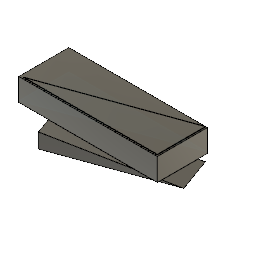
Pill holder for dispense v1 (Autodesk Fusion 360 design; units mm, degrees)
Autodesk Fusion 360 part; units mm, degrees
sketch "Sketch3" plane through (0, 0, 0) normal (0, 0, 1) x (1, 0, 0) in component "Pill Holder "
  line L0 (0, -3.5074) -> (3, -3.5074)
  line L1 (3, -3.5074) -> (3, 110.4926)
  line L2 (3, 110.4926) -> (0, 110.4926)
  line L3 (0, 110.4926) -> (0, -3.5074)
  dimension "d20" = 114
  dimension "d21" = 3
  constraint horizontal L0
  constraint vertical L1
  constraint horizontal L2
  constraint vertical L3
  measures "d20" distance of L0.end L1.end
  measures "d21" distance of L0.start L0.end
extrude "Extrude6" add sketch "Sketch3" along normal blind 50 makes body 1 in component "Pill Holder "
sketch "Sketch4" plane through (0, 0, 0) normal (-1, 0, 0) x (0, -1, 0) in component "Pill Holder "
  line L0 (-110.4926, 0) -> (3.5074, 0)
  line L1 (3.5074, 0) -> (3.5074, 50)
  line L2 (3.5074, 50) -> (-110.4926, 50)
  line L3 (-110.4926, 50) -> (-110.4926, 0)
  line L4 (0.5074, 3) -> (-107.4926, 3)
  line L5 (-107.4926, 3) -> (-107.4926, 47)
  line L6 (-107.4926, 47) -> (0.5074, 47)
  line L7 (0.5074, 47) -> (0.5074, 3)
  dimension "d24" = 3
  dimension "d25" = 3
  dimension "d26" = 3
  dimension "d27" = 3
  constraint horizontal L4
  constraint vertical L5
  constraint horizontal L6
  constraint vertical L7
  measures "d24" distance of L0 L4
  measures "d25" distance of L2 L6
  measures "d26" distance of L1 L7
  measures "d27" distance of L3 L5
extrude "Extrude7" add sketch "Sketch4" along normal blind 304 bodies 1 in component "Pill Holder "
extrude "Extrude8" cut 1 faces at (-201.6667, 110.4926, 16.6667) along direction (0, -1, 0) blind 3 on bodies 1 bodies 1 in component "Pill Holder "
sketch "Sketch5" plane through (0, 0, 3) normal (0, 0, 1) x (-1, 0, 0) in component "Pill Holder "
  line L0 (0, 0.5074) -> (0, -107.4926)
  line L1 (0, -107.4926) -> (304, -107.4926)
  line L2 (304, -107.4926) -> (304, 0.5074)
  line L3 (304, 0.5074) -> (0, 0.5074)
  line L4 (-3, -107.4926) -> (304, -107.4926)
  line L5 (304, -107.4926) -> (304, 3.5074)
  line L6 (304, 3.5074) -> (-3, 3.5074)
  line L7 (-3, 3.5074) -> (-3, -107.4926)
  line L8 (0, -107.4926) -> (0, 0.5074)
  line L9 (0, 0.5074) -> (304, 0.5074)
  line L10 (304, 0.5074) -> (304, -107.4926)
  line L11 (304, -107.4926) -> (0, -107.4926)
  line L12 (304, 3.5074) -> (-3, -107.4926)
  constraint coincident L5.end L6.start
  constraint coincident L4.start L7.end
extrude "Extrude11" add sketch "Sketch5" along normal blind 48 contours L0 L3 L8 L9 L12 bodies 1 in component "Pill Holder "
sketch "Sketch6" plane through (-304, 0, 0) normal (-1, 0, 0) x (0, -1, 0) in component "Pill Holder "
  line L0 (-107.4926, 50) -> (-107.4926, 47)
  line L1 (-107.4926, 47) -> (0.5074, 47)
  line L2 (0.5074, 3) -> (-107.4926, 3)
  line L3 (-107.4926, 0) -> (3.5074, 0)
  line L4 (3.5074, 0) -> (3.5074, 50)
  line L5 (3.5074, 50) -> (-107.4926, 50)
  line L6 (3.5074, 9.4187) -> (-98.3183, 50)
  line L7 (0.5074, 47) -> (0.5074, 3)
  line L8 (-107.4926, 3) -> (-107.4926, 0)
  constraint coincident L4 L6.start
  constraint coincident L5 L6.end
sketch "Sketch7" plane through (-34.0252, 94.1056, 0) normal (-0.340021, 0.940418, 0) x (-0.940418, -0.340021, 0) in component "Pill Holder "
  line L0 (278.2567, 47) -> (-36.1809, 47)
  line L1 (-36.1809, 47) -> (-36.1809, 3)
  line L2 (-36.1809, 3) -> (278.2567, 3)
  line L3 (278.2567, 3) -> (278.2567, 47)
  line L4 (52.2027, 3) -> (278.2567, 38.5389)
  constraint coincident L2 L4.start
  constraint coincident L3 L4.end
sketch "Sketch8" plane through (0, 0, 3) normal (0, 0, 1) x (-1, 0, 0) in component "Pill Holder "
  line L0 (295.7027, 0.5074) -> (0, -106.4079)
  line L1 (0, -106.4079) -> (0, -107.4926)
  line L2 (0, -107.4926) -> (304, -107.4926)
  line L3 (304, -107.4926) -> (304, 0.5074)
  line L4 (304, 0.5074) -> (295.7027, 0.5074)
sketch "Sketch1" plane through (-34.0252, 94.1056, 0) normal (-0.340021, 0.940418, 0) x (-0.940418, -0.340021, 0) in component "wal"
  line L0 (278.2567, 47) -> (-36.1809, 47)
  line L1 (-36.1809, 47) -> (-36.1809, 3)
  line L2 (-36.1809, 3) -> (278.2567, 3)
  line L3 (278.2567, 3) -> (278.2567, 47)
  line L4 (26.6613, 3) -> (278.2567, 36.0366)
  dimension "d44" = 253.7551
  constraint coincident L2 L4.start
  constraint coincident L3 L4.end
  measures "d44" distance of L4.start L4.end
extrude "Extrude1" add sketch "Sketch1" along normal blind 80 separate body contours L2 L3 L4 makes body 2 in component "wal"
component "Pill Holder " placed x (1, 0, 0) y (0, 1, 0) z (0, 0, 1) at (0.3608, 1.2387, 1.5611)
component "wal" placed x (1, 0, 0) y (0, 1, 0) z (0, 0, 1) at (0, 0, 0) in component "Pill Holder "
